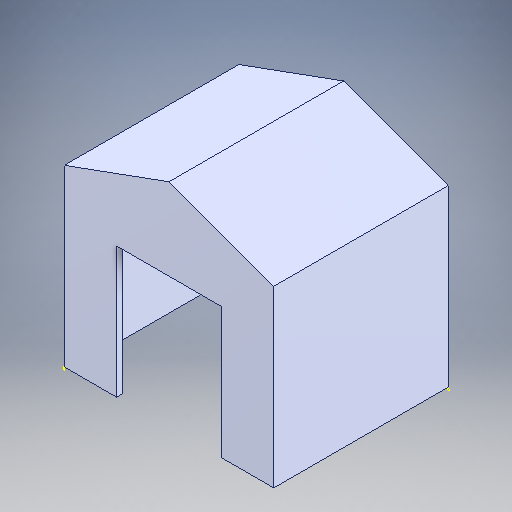
# Autodesk Inventor part: HCRO Shed_v0
Saved by Autodesk Inventor 2025.3 (Build 293356000, 356)
## iProperties
Created: 2025-10-31
Part Number: HCRO Shed_v0
Material: Generic
Description: STEP AP214
Document SubType Name: Modeling
Designer: sonata
Density: 1 g/cm^3
Appearance: Default
Sending System: SolidWorks 2024
Preprocessor: SwSTEP 2.0
Title: HCRO Shed_v0.STEP
Revision Number: ANY
Autodesk Inventor part; units mm, degrees
ref_plane "YZ Plane" through (0, 0, 0) normal (1, 0, 0) x (0, 1, 0)
ref_plane "XZ Plane" through (0, 0, 0) normal (0, 1, 0) x (-1, 0, 0)
ref_plane "XY Plane" through (0, 0, 0) normal (0, 0, 1) x (1, 0, 0)
ref_plane "Work Plane1" through (-1828.8, 0, 1524) normal (0, 1, 0) x (1, 0, 0)
sketch "Sketch13" plane through (-1828.8, 0, 1524) normal (0, 1, 0) x (1, 0, 0)
  line L0 (0, 0) -> (0, 3048) projected
  line L1 (0, 0) -> (914.4, 0)
  line L2 (3657.6, 0) -> (0, 0) projected
  line L3 (914.4, 101.6) -> (101.6, 101.6)
  line L4 (101.6, 101.6) -> (101.6, 2946.4)
  line L5 (101.6, 2946.4) -> (3556, 2946.4)
  line L6 (3556, 2946.4) -> (3556, 101.6)
  line L7 (3556, 101.6) -> (2743.2, 101.6)
  line L8 (2743.2, 101.6) -> (2743.2, 0)
  line L9 (914.4, 0) -> (914.4, 101.6)
  line L10 (3657.6, 3048) -> (3657.6, 0) projected
  line L11 (0, 3048) -> (3657.6, 3048) projected
  point P0 (1828.8, 1524)
  dimension "d25" = 101.6
  dimension "d26" = 914.4
  dimension "d27" = 101.6
  dimension "d28" = 101.6
  dimension "d29" = 101.6
  constraints: 16 end point, 4 perpendicular, 4 point on line, 1 collinear, 1 horizontal, 1 vertical
  measures "d25" distance of L1.end L3.start
  measures "d26" distance of L0.start L1.end
  measures "d27" distance between parallel lines of L10 L6
  measures "d28" distance between parallel lines of L0 L4
  measures "d29" distance between parallel lines of L11 L5
extrude "Extrusion9" add sketch "Sketch13" along normal blind 3048 contours L0 L11 L10 L2 L8 L7 L6 L5 L4 L3 L9 L1
ref_plane "Work Plane3" through (-1828.8, -38.1, 1524) normal (0, 0, 1) x (1, 0, 0)
sketch "Sketch14" plane through (-1828.8, -38.1, 1524) normal (0, 0, 1) x (1, 0, 0)
  line L0 (914.4, 38.1) -> (914.4, 3086.1) projected
  line L1 (914.4, 2324.1) -> (2743.2, 2324.1)
  line L2 (2743.2, 38.1) -> (2743.2, 3086.1) projected
  line L3 (2743.2, 38.1) -> (914.4, 38.1) projected
  line L4 (914.4, 3086.1) -> (2743.2, 3086.1)
  point P0 (1828.8, 38.1)
  dimension "d32" = 2286
  constraints: 4 end point, 2 horizontal, 2 point on line
  measures "d32" distance between parallel lines of L3 L1
extrude "Extrusion10" add sketch "Sketch14" against normal blind 101.6 contours L0 L4 L2 L1
ref_plane "Work Plane4" through (-1828.8, -38.1, 1524) normal (0, 0, 1) x (1, 0, 0)
sketch "Sketch15" plane through (-1828.8, -38.1, 1524) normal (0, 0, 1) x (1, 0, 0)
  line L0 (3657.6, 3086.1) -> (0, 3086.1) projected
  line L1 (0, 3086.1) -> (1828.8, 3751.5924)
  line L2 (1828.8, 3751.5924) -> (3657.6, 3086.1)
  point P0 (1828.8, 38.1)
  dimension "d35" = 19.996
  constraints: 4 end point, 1 equal length
  measures "d35" angle of L1 L0
extrude "Extrusion11" add sketch "Sketch15" against normal blind 101.6
ref_plane "Work Plane2" through (1828.8, -38.1, -1524) normal (0, 0, -1) x (-1, 0, 0)
sketch "Sketch17" plane through (1828.8, -38.1, -1524) normal (0, 0, -1) x (-1, 0, 0)
  line L0 (63.5, 3086.1) -> (0, 3086.1) projected
  line L1 (1828.8, 3751.5924) -> (0, 3086.1) projected
  line L2 (0, 3086.1) -> (1828.8, 3751.5924)
  line L3 (3657.6, 0) -> (3657.6, 3086.1) projected
  line L4 (1828.8, 3751.5924) -> (3657.6, 3086.1)
  line L5 (0, 3086.1) -> (3657.6, 3086.1)
  point P0 (1828.8, 38.1)
  constraints: 6 end point, 1 collinear, 1 horizontal
extrude "Extrusion12" add sketch "Sketch17" against normal blind 101.6
sketch "Sketch19" plane through (1828.8, 0, -1524) normal (0, 0, -1) x (-1, 0, 0)
  line L0 (0, 3048) -> (101.6, 3048) projected
  line L1 (0, 3048) -> (101.6, 3048)
  line L2 (101.6, 3048) -> (1828.8, 3676.5206)
  line L3 (3556, 0) -> (3556, 3048) projected
  line L4 (1828.8, 3676.5206) -> (3556, 3048)
  line L5 (1828.8, 3713.4924) -> (3657.6, 3048) projected
  line L6 (3556, 3048) -> (3657.6, 3048)
  line L7 (3657.6, 3048) -> (1828.8, 3713.4924)
  line L8 (1828.8, 3713.4924) -> (0, 3048)
  point P0 (1828.8, 0)
  constraints: 12 end point, 3 collinear, 2 parallel
extrude "Extrusion14" add sketch "Sketch19" against normal blind 3048
sketch "Sketch20" plane through (1828.8, 0, -1524) normal (0, 0, -1) x (-1, 0, 0)
  line L0 (228.6, 1270) -> (584.2, 1270)
  line L1 (584.2, 1270) -> (584.2, 965.2)
  line L2 (584.2, 965.2) -> (228.6, 965.2)
  line L3 (228.6, 965.2) -> (228.6, 1270)
  line L4 (0, 0) -> (0, 3048) projected
  line L5 (0, 0) -> (3657.6, 0) projected
  point P0 (1828.8, 0)
  point P1 (228.6, 1117.6)
  dimension "d44" = 228.6
  dimension "d45" = 355.6
  dimension "d46" = 304.8
  dimension "d47" = 965.2
  constraints: 8 end point, 2 parallel, 1 horizontal, 1 midpoint, 1 perpendicular
  measures "d44" distance between parallel lines of L4 L3
  measures "d45" distance from line of point (228.6, 1117.6) L1
  measures "d46" distance between parallel lines of L2 L0
  measures "d47" distance between parallel lines of L5 L2
extrude "Extrusion15" cut sketch "Sketch20" against normal blind 101.6
sketch "Sketch21" plane through (1828.8, 0, -1524) normal (0, 0, -1) x (-1, 0, 0)
  line L0 (1676.4, 3048) -> (1981.2, 3048)
  line L1 (1981.2, 3048) -> (1981.2, 2743.2)
  line L2 (1981.2, 2743.2) -> (1676.4, 2743.2)
  line L3 (1676.4, 2743.2) -> (1676.4, 3048)
  line L4 (3657.6, 3048) -> (1828.8, 3713.4924) projected
  line L5 (1828.8, 3713.4924) -> (1828.8, 2743.2) construction
  line L6 (0, 0) -> (0, 3048) projected
  line L7 (3657.6, 0) -> (3657.6, 3048) projected
  line L8 (0, 3048) -> (3657.6, 3048) construction
  point P0 (1828.8, 0)
  dimension "d50" = 304.8
  dimension "d51" = 304.8
  constraints: 12 end point, 2 horizontal, 2 parallel, 1 collinear, 1 midpoint, 1 perpendicular, 1 vertical
  measures "d50" distance of L0.start L0.end
  measures "d51" distance between parallel lines of L0 L2
extrude "Extrusion16" cut sketch "Sketch21" against normal blind 101.6
body "Solid1"
